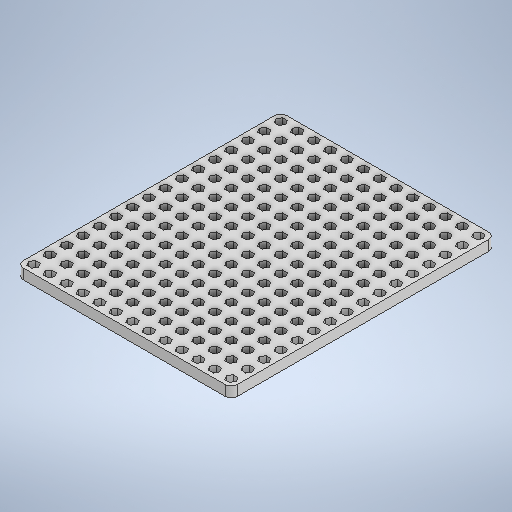
# Autodesk Inventor part: bottom
Saved by Autodesk Inventor 2025.1 (Build 291241000, 241)
## iProperties
Created: 2024-10-26
Part Number: bottom
Material: 일반
Document SubType Name: Sheet Metal
Designer: goode
Density: 1 g/cm^3
Sheet Metal Rule: 기본값_mm
Appearance: 기본값
Author: goode
Autodesk Inventor part; units mm, degrees
(part 1 of 2)
ref_plane "YZ Plane" through (0, 0, 0) normal (1, 0, 0) x (0, 1, 0)
ref_plane "XZ Plane" through (0, 0, 0) normal (0, 1, 0) x (-1, 0, 0)
ref_plane "XY Plane" through (0, 0, 0) normal (0, 0, 1) x (1, 0, 0)
sketch "스케치1" plane through (0, 0, 0) normal (0, 1, 0) x (-1, 0, 0)
  circle A0 centre (0, 0) radius 2.05
  line L0 (-1.1836, 2.05) -> (1.1836, 2.05)
  line L1 (1.1836, 2.05) -> (2.3671, 0)
  line L2 (2.3671, 0) -> (1.1836, -2.05)
  line L3 (1.1836, -2.05) -> (-1.1836, -2.05)
  line L4 (-1.1836, -2.05) -> (-2.3671, 0)
  line L5 (-2.3671, 0) -> (-1.1836, 2.05)
  circle A1 centre (0, 0) radius 1.1
  line L6 (-3, 0) -> (-3, 3)
  line L7 (-3, 3) -> (0, 3)
  circle A2 centre (0, -8) radius 2.05
  line L8 (-1.1836, -5.95) -> (1.1836, -5.95)
  line L9 (1.1836, -5.95) -> (2.3671, -8)
  line L10 (2.3671, -8) -> (1.1836, -10.05)
  line L11 (1.1836, -10.05) -> (-1.1836, -10.05)
  line L12 (-1.1836, -10.05) -> (-2.3671, -8)
  line L13 (-2.3671, -8) -> (-1.1836, -5.95)
  circle A3 centre (0, -8) radius 1.1
  circle A4 centre (0, -16) radius 2.05
  line L14 (-1.1836, -13.95) -> (1.1836, -13.95)
  line L15 (1.1836, -13.95) -> (2.3671, -16)
  line L16 (2.3671, -16) -> (1.1836, -18.05)
  line L17 (1.1836, -18.05) -> (-1.1836, -18.05)
  line L18 (-1.1836, -18.05) -> (-2.3671, -16)
  line L19 (-2.3671, -16) -> (-1.1836, -13.95)
  circle A5 centre (0, -16) radius 1.1
  circle A6 centre (0, -24) radius 2.05
  line L20 (-1.1836, -21.95) -> (1.1836, -21.95)
  line L21 (1.1836, -21.95) -> (2.3671, -24)
  line L22 (2.3671, -24) -> (1.1836, -26.05)
  line L23 (1.1836, -26.05) -> (-1.1836, -26.05)
  line L24 (-1.1836, -26.05) -> (-2.3671, -24)
  line L25 (-2.3671, -24) -> (-1.1836, -21.95)
  circle A7 centre (0, -24) radius 1.1
  circle A8 centre (0, -32) radius 2.05
  line L26 (-1.1836, -29.95) -> (1.1836, -29.95)
  line L27 (1.1836, -29.95) -> (2.3671, -32)
  line L28 (2.3671, -32) -> (1.1836, -34.05)
  line L29 (1.1836, -34.05) -> (-1.1836, -34.05)
  line L30 (-1.1836, -34.05) -> (-2.3671, -32)
  line L31 (-2.3671, -32) -> (-1.1836, -29.95)
  circle A9 centre (0, -32) radius 1.1
  circle A10 centre (0, -40) radius 2.05
  line L32 (-1.1836, -37.95) -> (1.1836, -37.95)
  line L33 (1.1836, -37.95) -> (2.3671, -40)
  line L34 (2.3671, -40) -> (1.1836, -42.05)
  line L35 (1.1836, -42.05) -> (-1.1836, -42.05)
  line L36 (-1.1836, -42.05) -> (-2.3671, -40)
  line L37 (-2.3671, -40) -> (-1.1836, -37.95)
  circle A11 centre (0, -40) radius 1.1
  circle A12 centre (0, -48) radius 2.05
  line L38 (-1.1836, -45.95) -> (1.1836, -45.95)
  line L39 (1.1836, -45.95) -> (2.3671, -48)
  line L40 (2.3671, -48) -> (1.1836, -50.05)
  line L41 (1.1836, -50.05) -> (-1.1836, -50.05)
  line L42 (-1.1836, -50.05) -> (-2.3671, -48)
  line L43 (-2.3671, -48) -> (-1.1836, -45.95)
  circle A13 centre (0, -48) radius 1.1
  circle A14 centre (0, -56) radius 2.05
  line L44 (-1.1836, -53.95) -> (1.1836, -53.95)
  line L45 (1.1836, -53.95) -> (2.3671, -56)
  line L46 (2.3671, -56) -> (1.1836, -58.05)
  line L47 (1.1836, -58.05) -> (-1.1836, -58.05)
  line L48 (-1.1836, -58.05) -> (-2.3671, -56)
  line L49 (-2.3671, -56) -> (-1.1836, -53.95)
  circle A15 centre (0, -56) radius 1.1
  circle A16 centre (0, -64) radius 2.05
  line L50 (-1.1836, -61.95) -> (1.1836, -61.95)
  line L51 (1.1836, -61.95) -> (2.3671, -64)
  line L52 (2.3671, -64) -> (1.1836, -66.05)
  line L53 (1.1836, -66.05) -> (-1.1836, -66.05)
  line L54 (-1.1836, -66.05) -> (-2.3671, -64)
  line L55 (-2.3671, -64) -> (-1.1836, -61.95)
  circle A17 centre (0, -64) radius 1.1
  circle A18 centre (0, -72) radius 2.05
  line L56 (-1.1836, -69.95) -> (1.1836, -69.95)
  line L57 (1.1836, -69.95) -> (2.3671, -72)
  line L58 (2.3671, -72) -> (1.1836, -74.05)
  line L59 (1.1836, -74.05) -> (-1.1836, -74.05)
  line L60 (-1.1836, -74.05) -> (-2.3671, -72)
  line L61 (-2.3671, -72) -> (-1.1836, -69.95)
  circle A19 centre (0, -72) radius 1.1
  circle A20 centre (0, -80) radius 2.05
  line L62 (-1.1836, -77.95) -> (1.1836, -77.95)
  line L63 (1.1836, -77.95) -> (2.3671, -80)
  line L64 (2.3671, -80) -> (1.1836, -82.05)
  line L65 (1.1836, -82.05) -> (-1.1836, -82.05)
  line L66 (-1.1836, -82.05) -> (-2.3671, -80)
  line L67 (-2.3671, -80) -> (-1.1836, -77.95)
  circle A21 centre (0, -80) radius 1.1
  circle A22 centre (0, -88) radius 2.05
  line L68 (-1.1836, -85.95) -> (1.1836, -85.95)
  line L69 (1.1836, -85.95) -> (2.3671, -88)
  line L70 (2.3671, -88) -> (1.1836, -90.05)
  line L71 (1.1836, -90.05) -> (-1.1836, -90.05)
  line L72 (-1.1836, -90.05) -> (-2.3671, -88)
  line L73 (-2.3671, -88) -> (-1.1836, -85.95)
  circle A23 centre (0, -88) radius 1.1
  circle A24 centre (0, -96) radius 2.05
  line L74 (-1.1836, -93.95) -> (1.1836, -93.95)
  line L75 (1.1836, -93.95) -> (2.3671, -96)
  line L76 (2.3671, -96) -> (1.1836, -98.05)
  line L77 (1.1836, -98.05) -> (-1.1836, -98.05)
  line L78 (-1.1836, -98.05) -> (-2.3671, -96)
  line L79 (-2.3671, -96) -> (-1.1836, -93.95)
  circle A25 centre (0, -96) radius 1.1
  circle A26 centre (0, -104) radius 2.05
  line L80 (-1.1836, -101.95) -> (1.1836, -101.95)
  line L81 (1.1836, -101.95) -> (2.3671, -104)
  line L82 (2.3671, -104) -> (1.1836, -106.05)
  line L83 (1.1836, -106.05) -> (-1.1836, -106.05)
  line L84 (-1.1836, -106.05) -> (-2.3671, -104)
  line L85 (-2.3671, -104) -> (-1.1836, -101.95)
  circle A27 centre (0, -104) radius 1.1
  circle A28 centre (0, -112) radius 2.05
  line L86 (-1.1836, -109.95) -> (1.1836, -109.95)
  line L87 (1.1836, -109.95) -> (2.3671, -112)
  line L88 (2.3671, -112) -> (1.1836, -114.05)
  line L89 (1.1836, -114.05) -> (-1.1836, -114.05)
  line L90 (-1.1836, -114.05) -> (-2.3671, -112)
  line L91 (-2.3671, -112) -> (-1.1836, -109.95)
  circle A29 centre (0, -112) radius 1.1
  circle A30 centre (0, -120) radius 2.05
  line L92 (-1.1836, -117.95) -> (1.1836, -117.95)
  line L93 (1.1836, -117.95) -> (2.3671, -120)
  line L94 (2.3671, -120) -> (1.1836, -122.05)
  line L95 (1.1836, -122.05) -> (-1.1836, -122.05)
  line L96 (-1.1836, -122.05) -> (-2.3671, -120)
  line L97 (-2.3671, -120) -> (-1.1836, -117.95)
  circle A31 centre (0, -120) radius 1.1
  circle A32 centre (8, 0) radius 2.05
  line L98 (6.8164, 2.05) -> (9.1836, 2.05)
  line L99 (9.1836, 2.05) -> (10.3671, 0)
  line L100 (10.3671, 0) -> (9.1836, -2.05)
  line L101 (9.1836, -2.05) -> (6.8164, -2.05)
  line L102 (6.8164, -2.05) -> (5.6329, 0)
  line L103 (5.6329, 0) -> (6.8164, 2.05)
  circle A33 centre (8, 0) radius 1.1
  circle A34 centre (8, -8) radius 2.05
  line L104 (6.8164, -5.95) -> (9.1836, -5.95)
  line L105 (9.1836, -5.95) -> (10.3671, -8)
  line L106 (10.3671, -8) -> (9.1836, -10.05)
  line L107 (9.1836, -10.05) -> (6.8164, -10.05)
  line L108 (6.8164, -10.05) -> (5.6329, -8)
  line L109 (5.6329, -8) -> (6.8164, -5.95)
  circle A35 centre (8, -8) radius 1.1
  circle A36 centre (8, -16) radius 2.05
  line L110 (6.8164, -13.95) -> (9.1836, -13.95)
  line L111 (9.1836, -13.95) -> (10.3671, -16)
  line L112 (10.3671, -16) -> (9.1836, -18.05)
  line L113 (9.1836, -18.05) -> (6.8164, -18.05)
  line L114 (6.8164, -18.05) -> (5.6329, -16)
  line L115 (5.6329, -16) -> (6.8164, -13.95)
  circle A37 centre (8, -16) radius 1.1
  circle A38 centre (8, -24) radius 2.05
  line L116 (6.8164, -21.95) -> (9.1836, -21.95)
  line L117 (9.1836, -21.95) -> (10.3671, -24)
  line L118 (10.3671, -24) -> (9.1836, -26.05)
  line L119 (9.1836, -26.05) -> (6.8164, -26.05)
  line L120 (6.8164, -26.05) -> (5.6329, -24)
  line L121 (5.6329, -24) -> (6.8164, -21.95)
  circle A39 centre (8, -24) radius 1.1
  circle A40 centre (8, -32) radius 2.05
  line L122 (6.8164, -29.95) -> (9.1836, -29.95)
  line L123 (9.1836, -29.95) -> (10.3671, -32)
  line L124 (10.3671, -32) -> (9.1836, -34.05)
  line L125 (9.1836, -34.05) -> (6.8164, -34.05)
  line L126 (6.8164, -34.05) -> (5.6329, -32)
  line L127 (5.6329, -32) -> (6.8164, -29.95)
  circle A41 centre (8, -32) radius 1.1
  circle A42 centre (8, -40) radius 2.05
  line L128 (6.8164, -37.95) -> (9.1836, -37.95)
  line L129 (9.1836, -37.95) -> (10.3671, -40)
  line L130 (10.3671, -40) -> (9.1836, -42.05)
  line L131 (9.1836, -42.05) -> (6.8164, -42.05)
  line L132 (6.8164, -42.05) -> (5.6329, -40)
  line L133 (5.6329, -40) -> (6.8164, -37.95)
  circle A43 centre (8, -40) radius 1.1
  circle A44 centre (8, -48) radius 2.05
  line L134 (6.8164, -45.95) -> (9.1836, -45.95)
  line L135 (9.1836, -45.95) -> (10.3671, -48)
  line L136 (10.3671, -48) -> (9.1836, -50.05)
  line L137 (9.1836, -50.05) -> (6.8164, -50.05)
  line L138 (6.8164, -50.05) -> (5.6329, -48)
  line L139 (5.6329, -48) -> (6.8164, -45.95)
  circle A45 centre (8, -48) radius 1.1
  circle A46 centre (8, -56) radius 2.05
  line L140 (6.8164, -53.95) -> (9.1836, -53.95)
  line L141 (9.1836, -53.95) -> (10.3671, -56)
  line L142 (10.3671, -56) -> (9.1836, -58.05)
  line L143 (9.1836, -58.05) -> (6.8164, -58.05)
  line L144 (6.8164, -58.05) -> (5.6329, -56)
  line L145 (5.6329, -56) -> (6.8164, -53.95)
  circle A47 centre (8, -56) radius 1.1
  circle A48 centre (8, -64) radius 2.05
  line L146 (6.8164, -61.95) -> (9.1836, -61.95)
  line L147 (9.1836, -61.95) -> (10.3671, -64)
  line L148 (10.3671, -64) -> (9.1836, -66.05)
  line L149 (9.1836, -66.05) -> (6.8164, -66.05)
  line L150 (6.8164, -66.05) -> (5.6329, -64)
  line L151 (5.6329, -64) -> (6.8164, -61.95)
  circle A49 centre (8, -64) radius 1.1
  circle A50 centre (8, -72) radius 2.05
  line L152 (6.8164, -69.95) -> (9.1836, -69.95)
  line L153 (9.1836, -69.95) -> (10.3671, -72)
  line L154 (10.3671, -72) -> (9.1836, -74.05)
  line L155 (9.1836, -74.05) -> (6.8164, -74.05)
  line L156 (6.8164, -74.05) -> (5.6329, -72)
  line L157 (5.6329, -72) -> (6.8164, -69.95)
  circle A51 centre (8, -72) radius 1.1
  circle A52 centre (8, -80) radius 2.05
  line L158 (6.8164, -77.95) -> (9.1836, -77.95)
  line L159 (9.1836, -77.95) -> (10.3671, -80)
  line L160 (10.3671, -80) -> (9.1836, -82.05)
  line L161 (9.1836, -82.05) -> (6.8164, -82.05)
  line L162 (6.8164, -82.05) -> (5.6329, -80)
  line L163 (5.6329, -80) -> (6.8164, -77.95)
  circle A53 centre (8, -80) radius 1.1
  circle A54 centre (8, -88) radius 2.05
  line L164 (6.8164, -85.95) -> (9.1836, -85.95)
  line L165 (9.1836, -85.95) -> (10.3671, -88)
  line L166 (10.3671, -88) -> (9.1836, -90.05)
  line L167 (9.1836, -90.05) -> (6.8164, -90.05)
  line L168 (6.8164, -90.05) -> (5.6329, -88)
  line L169 (5.6329, -88) -> (6.8164, -85.95)
  circle A55 centre (8, -88) radius 1.1
  circle A56 centre (8, -96) radius 2.05
  line L170 (6.8164, -93.95) -> (9.1836, -93.95)
  line L171 (9.1836, -93.95) -> (10.3671, -96)
  line L172 (10.3671, -96) -> (9.1836, -98.05)
  line L173 (9.1836, -98.05) -> (6.8164, -98.05)
  line L174 (6.8164, -98.05) -> (5.6329, -96)
  line L175 (5.6329, -96) -> (6.8164, -93.95)
  circle A57 centre (8, -96) radius 1.1
  circle A58 centre (8, -104) radius 2.05
  line L176 (6.8164, -101.95) -> (9.1836, -101.95)
  line L177 (9.1836, -101.95) -> (10.3671, -104)
  line L178 (10.3671, -104) -> (9.1836, -106.05)
  line L179 (9.1836, -106.05) -> (6.8164, -106.05)
  line L180 (6.8164, -106.05) -> (5.6329, -104)
  line L181 (5.6329, -104) -> (6.8164, -101.95)
  circle A59 centre (8, -104) radius 1.1
  circle A60 centre (8, -112) radius 2.05
  line L182 (6.8164, -109.95) -> (9.1836, -109.95)
  line L183 (9.1836, -109.95) -> (10.3671, -112)
  line L184 (10.3671, -112) -> (9.1836, -114.05)
  line L185 (9.1836, -114.05) -> (6.8164, -114.05)
  line L186 (6.8164, -114.05) -> (5.6329, -112)
  line L187 (5.6329, -112) -> (6.8164, -109.95)
  circle A61 centre (8, -112) radius 1.1
  circle A62 centre (8, -120) radius 2.05
  line L188 (6.8164, -117.95) -> (9.1836, -117.95)
  line L189 (9.1836, -117.95) -> (10.3671, -120)
  line L190 (10.3671, -120) -> (9.1836, -122.05)
  line L191 (9.1836, -122.05) -> (6.8164, -122.05)
  line L192 (6.8164, -122.05) -> (5.6329, -120)
  line L193 (5.6329, -120) -> (6.8164, -117.95)
  circle A63 centre (8, -120) radius 1.1
  circle A64 centre (16, 0) radius 2.05
  line L194 (14.8164, 2.05) -> (17.1836, 2.05)
  line L195 (17.1836, 2.05) -> (18.3671, 0)
  line L196 (18.3671, 0) -> (17.1836, -2.05)
  line L197 (17.1836, -2.05) -> (14.8164, -2.05)
  line L198 (14.8164, -2.05) -> (13.6329, 0)
  line L199 (13.6329, 0) -> (14.8164, 2.05)
  circle A65 centre (16, 0) radius 1.1
  circle A66 centre (16, -8) radius 2.05
  line L200 (14.8164, -5.95) -> (17.1836, -5.95)
  line L201 (17.1836, -5.95) -> (18.3671, -8)
  line L202 (18.3671, -8) -> (17.1836, -10.05)
  line L203 (17.1836, -10.05) -> (14.8164, -10.05)
  line L204 (14.8164, -10.05) -> (13.6329, -8)
  line L205 (13.6329, -8) -> (14.8164, -5.95)
  circle A67 centre (16, -8) radius 1.1
  circle A68 centre (16, -16) radius 2.05
  line L206 (14.8164, -13.95) -> (17.1836, -13.95)
  line L207 (17.1836, -13.95) -> (18.3671, -16)
  line L208 (18.3671, -16) -> (17.1836, -18.05)
  line L209 (17.1836, -18.05) -> (14.8164, -18.05)
  line L210 (14.8164, -18.05) -> (13.6329, -16)
  line L211 (13.6329, -16) -> (14.8164, -13.95)
  circle A69 centre (16, -16) radius 1.1
  circle A70 centre (16, -24) radius 2.05
  line L212 (14.8164, -21.95) -> (17.1836, -21.95)
  line L213 (17.1836, -21.95) -> (18.3671, -24)
  line L214 (18.3671, -24) -> (17.1836, -26.05)
  line L215 (17.1836, -26.05) -> (14.8164, -26.05)
  line L216 (14.8164, -26.05) -> (13.6329, -24)
  line L217 (13.6329, -24) -> (14.8164, -21.95)
  circle A71 centre (16, -24) radius 1.1
  circle A72 centre (16, -32) radius 2.05
  line L218 (14.8164, -29.95) -> (17.1836, -29.95)
  line L219 (17.1836, -29.95) -> (18.3671, -32)
  line L220 (18.3671, -32) -> (17.1836, -34.05)
  line L221 (17.1836, -34.05) -> (14.8164, -34.05)
  line L222 (14.8164, -34.05) -> (13.6329, -32)
  line L223 (13.6329, -32) -> (14.8164, -29.95)
  circle A73 centre (16, -32) radius 1.1
  circle A74 centre (16, -40) radius 2.05
  line L224 (14.8164, -37.95) -> (17.1836, -37.95)
  line L225 (17.1836, -37.95) -> (18.3671, -40)
  line L226 (18.3671, -40) -> (17.1836, -42.05)
  line L227 (17.1836, -42.05) -> (14.8164, -42.05)
  line L228 (14.8164, -42.05) -> (13.6329, -40)
  line L229 (13.6329, -40) -> (14.8164, -37.95)
  circle A75 centre (16, -40) radius 1.1
  circle A76 centre (16, -48) radius 2.05
  line L230 (14.8164, -45.95) -> (17.1836, -45.95)
  line L231 (17.1836, -45.95) -> (18.3671, -48)
  line L232 (18.3671, -48) -> (17.1836, -50.05)
  line L233 (17.1836, -50.05) -> (14.8164, -50.05)
  line L234 (14.8164, -50.05) -> (13.6329, -48)
  line L235 (13.6329, -48) -> (14.8164, -45.95)
  circle A77 centre (16, -48) radius 1.1
  circle A78 centre (16, -56) radius 2.05
  line L236 (14.8164, -53.95) -> (17.1836, -53.95)
  line L237 (17.1836, -53.95) -> (18.3671, -56)
  line L238 (18.3671, -56) -> (17.1836, -58.05)
  line L239 (17.1836, -58.05) -> (14.8164, -58.05)
  line L240 (14.8164, -58.05) -> (13.6329, -56)
  line L241 (13.6329, -56) -> (14.8164, -53.95)
  circle A79 centre (16, -56) radius 1.1
  circle A80 centre (16, -64) radius 2.05
  line L242 (14.8164, -61.95) -> (17.1836, -61.95)
  line L243 (17.1836, -61.95) -> (18.3671, -64)
  line L244 (18.3671, -64) -> (17.1836, -66.05)
  line L245 (17.1836, -66.05) -> (14.8164, -66.05)
  line L246 (14.8164, -66.05) -> (13.6329, -64)
  line L247 (13.6329, -64) -> (14.8164, -61.95)
  circle A81 centre (16, -64) radius 1.1
  circle A82 centre (16, -72) radius 2.05
  line L248 (14.8164, -69.95) -> (17.1836, -69.95)
  line L249 (17.1836, -69.95) -> (18.3671, -72)
  line L250 (18.3671, -72) -> (17.1836, -74.05)
  line L251 (17.1836, -74.05) -> (14.8164, -74.05)
  line L252 (14.8164, -74.05) -> (13.6329, -72)
  line L253 (13.6329, -72) -> (14.8164, -69.95)
  circle A83 centre (16, -72) radius 1.1
  circle A84 centre (16, -80) radius 2.05
  line L254 (14.8164, -77.95) -> (17.1836, -77.95)
  line L255 (17.1836, -77.95) -> (18.3671, -80)
  line L256 (18.3671, -80) -> (17.1836, -82.05)
  line L257 (17.1836, -82.05) -> (14.8164, -82.05)
  line L258 (14.8164, -82.05) -> (13.6329, -80)
  line L259 (13.6329, -80) -> (14.8164, -77.95)
  circle A85 centre (16, -80) radius 1.1
  circle A86 centre (16, -88) radius 2.05
  line L260 (14.8164, -85.95) -> (17.1836, -85.95)
  line L261 (17.1836, -85.95) -> (18.3671, -88)
  line L262 (18.3671, -88) -> (17.1836, -90.05)
  line L263 (17.1836, -90.05) -> (14.8164, -90.05)
  line L264 (14.8164, -90.05) -> (13.6329, -88)
  line L265 (13.6329, -88) -> (14.8164, -85.95)
  circle A87 centre (16, -88) radius 1.1
  circle A88 centre (16, -96) radius 2.05
  line L266 (14.8164, -93.95) -> (17.1836, -93.95)
  line L267 (17.1836, -93.95) -> (18.3671, -96)
  line L268 (18.3671, -96) -> (17.1836, -98.05)
  line L269 (17.1836, -98.05) -> (14.8164, -98.05)
  line L270 (14.8164, -98.05) -> (13.6329, -96)
  line L271 (13.6329, -96) -> (14.8164, -93.95)
  circle A89 centre (16, -96) radius 1.1
  circle A90 centre (16, -104) radius 2.05
  line L272 (14.8164, -101.95) -> (17.1836, -101.95)
  line L273 (17.1836, -101.95) -> (18.3671, -104)
  line L274 (18.3671, -104) -> (17.1836, -106.05)
  line L275 (17.1836, -106.05) -> (14.8164, -106.05)
  line L276 (14.8164, -106.05) -> (13.6329, -104)
  line L277 (13.6329, -104) -> (14.8164, -101.95)
  circle A91 centre (16, -104) radius 1.1
  circle A92 centre (16, -112) radius 2.05
  line L278 (14.8164, -109.95) -> (17.1836, -109.95)
  line L279 (17.1836, -109.95) -> (18.3671, -112)
  line L280 (18.3671, -112) -> (17.1836, -114.05)
  line L281 (17.1836, -114.05) -> (14.8164, -114.05)
  line L282 (14.8164, -114.05) -> (13.6329, -112)
  line L283 (13.6329, -112) -> (14.8164, -109.95)
  circle A93 centre (16, -112) radius 1.1
  circle A94 centre (16, -120) radius 2.05
  line L284 (14.8164, -117.95) -> (17.1836, -117.95)
  line L285 (17.1836, -117.95) -> (18.3671, -120)
  line L286 (18.3671, -120) -> (17.1836, -122.05)
  line L287 (17.1836, -122.05) -> (14.8164, -122.05)
  line L288 (14.8164, -122.05) -> (13.6329, -120)
  line L289 (13.6329, -120) -> (14.8164, -117.95)
  circle A95 centre (16, -120) radius 1.1
  circle A96 centre (24, 0) radius 2.05
  line L290 (22.8164, 2.05) -> (25.1836, 2.05)
  line L291 (25.1836, 2.05) -> (26.3671, 0)
  line L292 (26.3671, 0) -> (25.1836, -2.05)
  line L293 (25.1836, -2.05) -> (22.8164, -2.05)
  line L294 (22.8164, -2.05) -> (21.6329, 0)
  line L295 (21.6329, 0) -> (22.8164, 2.05)
  circle A97 centre (24, 0) radius 1.1
  circle A98 centre (24, -8) radius 2.05
  line L296 (22.8164, -5.95) -> (25.1836, -5.95)
  line L297 (25.1836, -5.95) -> (26.3671, -8)
  line L298 (26.3671, -8) -> (25.1836, -10.05)
  line L299 (25.1836, -10.05) -> (22.8164, -10.05)
  line L300 (22.8164, -10.05) -> (21.6329, -8)
  line L301 (21.6329, -8) -> (22.8164, -5.95)
  circle A99 centre (24, -8) radius 1.1
  circle A100 centre (24, -16) radius 2.05
  line L302 (22.8164, -13.95) -> (25.1836, -13.95)
  line L303 (25.1836, -13.95) -> (26.3671, -16)
  line L304 (26.3671, -16) -> (25.1836, -18.05)
  line L305 (25.1836, -18.05) -> (22.8164, -18.05)
  line L306 (22.8164, -18.05) -> (21.6329, -16)
  line L307 (21.6329, -16) -> (22.8164, -13.95)
  circle A101 centre (24, -16) radius 1.1
  circle A102 centre (24, -24) radius 2.05
  line L308 (22.8164, -21.95) -> (25.1836, -21.95)
  line L309 (25.1836, -21.95) -> (26.3671, -24)
  line L310 (26.3671, -24) -> (25.1836, -26.05)
  line L311 (25.1836, -26.05) -> (22.8164, -26.05)
  line L312 (22.8164, -26.05) -> (21.6329, -24)
  line L313 (21.6329, -24) -> (22.8164, -21.95)
  circle A103 centre (24, -24) radius 1.1
  circle A104 centre (24, -32) radius 2.05
  line L314 (22.8164, -29.95) -> (25.1836, -29.95)
  line L315 (25.1836, -29.95) -> (26.3671, -32)
  line L316 (26.3671, -32) -> (25.1836, -34.05)
  line L317 (25.1836, -34.05) -> (22.8164, -34.05)
  line L318 (22.8164, -34.05) -> (21.6329, -32)
  line L319 (21.6329, -32) -> (22.8164, -29.95)
  circle A105 centre (24, -32) radius 1.1
  circle A106 centre (24, -40) radius 2.05
  line L320 (22.8164, -37.95) -> (25.1836, -37.95)
  line L321 (25.1836, -37.95) -> (26.3671, -40)
  line L322 (26.3671, -40) -> (25.1836, -42.05)
  line L323 (25.1836, -42.05) -> (22.8164, -42.05)
  line L324 (22.8164, -42.05) -> (21.6329, -40)
  line L325 (21.6329, -40) -> (22.8164, -37.95)
  circle A107 centre (24, -40) radius 1.1
  circle A108 centre (24, -48) radius 2.05
  line L326 (22.8164, -45.95) -> (25.1836, -45.95)
  line L327 (25.1836, -45.95) -> (26.3671, -48)
  line L328 (26.3671, -48) -> (25.1836, -50.05)
  line L329 (25.1836, -50.05) -> (22.8164, -50.05)
  line L330 (22.8164, -50.05) -> (21.6329, -48)
  line L331 (21.6329, -48) -> (22.8164, -45.95)
  circle A109 centre (24, -48) radius 1.1
  circle A110 centre (24, -56) radius 2.05
  line L332 (22.8164, -53.95) -> (25.1836, -53.95)
  line L333 (25.1836, -53.95) -> (26.3671, -56)
  line L334 (26.3671, -56) -> (25.1836, -58.05)
  line L335 (25.1836, -58.05) -> (22.8164, -58.05)
  line L336 (22.8164, -58.05) -> (21.6329, -56)
  line L337 (21.6329, -56) -> (22.8164, -53.95)
  circle A111 centre (24, -56) radius 1.1
  circle A112 centre (24, -64) radius 2.05
  line L338 (22.8164, -61.95) -> (25.1836, -61.95)
  line L339 (25.1836, -61.95) -> (26.3671, -64)
  line L340 (26.3671, -64) -> (25.1836, -66.05)
  line L341 (25.1836, -66.05) -> (22.8164, -66.05)
  line L342 (22.8164, -66.05) -> (21.6329, -64)
  line L343 (21.6329, -64) -> (22.8164, -61.95)
  circle A113 centre (24, -64) radius 1.1
  circle A114 centre (24, -72) radius 2.05
  line L344 (22.8164, -69.95) -> (25.1836, -69.95)
  line L345 (25.1836, -69.95) -> (26.3671, -72)
  line L346 (26.3671, -72) -> (25.1836, -74.05)
  line L347 (25.1836, -74.05) -> (22.8164, -74.05)
  line L348 (22.8164, -74.05) -> (21.6329, -72)
  line L349 (21.6329, -72) -> (22.8164, -69.95)
  circle A115 centre (24, -72) radius 1.1
  circle A116 centre (24, -80) radius 2.05
  line L350 (22.8164, -77.95) -> (25.1836, -77.95)
  line L351 (25.1836, -77.95) -> (26.3671, -80)
  line L352 (26.3671, -80) -> (25.1836, -82.05)
  line L353 (25.1836, -82.05) -> (22.8164, -82.05)
  line L354 (22.8164, -82.05) -> (21.6329, -80)
  line L355 (21.6329, -80) -> (22.8164, -77.95)
  circle A117 centre (24, -80) radius 1.1
  circle A118 centre (24, -88) radius 2.05
  line L356 (22.8164, -85.95) -> (25.1836, -85.95)
  line L357 (25.1836, -85.95) -> (26.3671, -88)
  line L358 (26.3671, -88) -> (25.1836, -90.05)
  line L359 (25.1836, -90.05) -> (22.8164, -90.05)
  line L360 (22.8164, -90.05) -> (21.6329, -88)
  line L361 (21.6329, -88) -> (22.8164, -85.95)
  circle A119 centre (24, -88) radius 1.1
  circle A120 centre (24, -96) radius 2.05
  line L362 (22.8164, -93.95) -> (25.1836, -93.95)
  line L363 (25.1836, -93.95) -> (26.3671, -96)
  line L364 (26.3671, -96) -> (25.1836, -98.05)
  line L365 (25.1836, -98.05) -> (22.8164, -98.05)
  line L366 (22.8164, -98.05) -> (21.6329, -96)
  line L367 (21.6329, -96) -> (22.8164, -93.95)
  circle A121 centre (24, -96) radius 1.1
  circle A122 centre (24, -104) radius 2.05
  line L368 (22.8164, -101.95) -> (25.1836, -101.95)
  line L369 (25.1836, -101.95) -> (26.3671, -104)
  line L370 (26.3671, -104) -> (25.1836, -106.05)
  line L371 (25.1836, -106.05) -> (22.8164, -106.05)
  line L372 (22.8164, -106.05) -> (21.6329, -104)
  line L373 (21.6329, -104) -> (22.8164, -101.95)
  circle A123 centre (24, -104) radius 1.1
  circle A124 centre (24, -112) radius 2.05
  line L374 (22.8164, -109.95) -> (25.1836, -109.95)
  line L375 (25.1836, -109.95) -> (26.3671, -112)
  line L376 (26.3671, -112) -> (25.1836, -114.05)
  line L377 (25.1836, -114.05) -> (22.8164, -114.05)
  line L378 (22.8164, -114.05) -> (21.6329, -112)
  line L379 (21.6329, -112) -> (22.8164, -109.95)
  circle A125 centre (24, -112) radius 1.1
  circle A126 centre (24, -120) radius 2.05
  line L380 (22.8164, -117.95) -> (25.1836, -117.95)
  line L381 (25.1836, -117.95) -> (26.3671, -120)
  line L382 (26.3671, -120) -> (25.1836, -122.05)
  line L383 (25.1836, -122.05) -> (22.8164, -122.05)
  line L384 (22.8164, -122.05) -> (21.6329, -120)
  line L385 (21.6329, -120) -> (22.8164, -117.95)
  circle A127 centre (24, -120) radius 1.1
  circle A128 centre (32, 0) radius 2.05
  line L386 (30.8164, 2.05) -> (33.1836, 2.05)
  line L387 (33.1836, 2.05) -> (34.3671, 0)
  line L388 (34.3671, 0) -> (33.1836, -2.05)
  line L389 (33.1836, -2.05) -> (30.8164, -2.05)
  line L390 (30.8164, -2.05) -> (29.6329, 0)
  line L391 (29.6329, 0) -> (30.8164, 2.05)
  circle A129 centre (32, 0) radius 1.1
  circle A130 centre (32, -8) radius 2.05
  line L392 (30.8164, -5.95) -> (33.1836, -5.95)
  line L393 (33.1836, -5.95) -> (34.3671, -8)
  line L394 (34.3671, -8) -> (33.1836, -10.05)
  line L395 (33.1836, -10.05) -> (30.8164, -10.05)
  line L396 (30.8164, -10.05) -> (29.6329, -8)
  line L397 (29.6329, -8) -> (30.8164, -5.95)
  circle A131 centre (32, -8) radius 1.1
  circle A132 centre (32, -16) radius 2.05
  line L398 (30.8164, -13.95) -> (33.1836, -13.95)
  line L399 (33.1836, -13.95) -> (34.3671, -16)
  line L400 (34.3671, -16) -> (33.1836, -18.05)
  line L401 (33.1836, -18.05) -> (30.8164, -18.05)
  line L402 (30.8164, -18.05) -> (29.6329, -16)
  line L403 (29.6329, -16) -> (30.8164, -13.95)
  circle A133 centre (32, -16) radius 1.1
  circle A134 centre (32, -24) radius 2.05
  line L404 (30.8164, -21.95) -> (33.1836, -21.95)
  line L405 (33.1836, -21.95) -> (34.3671, -24)
  line L406 (34.3671, -24) -> (33.1836, -26.05)
  line L407 (33.1836, -26.05) -> (30.8164, -26.05)
  line L408 (30.8164, -26.05) -> (29.6329, -24)
  line L409 (29.6329, -24) -> (30.8164, -21.95)
  circle A135 centre (32, -24) radius 1.1
  circle A136 centre (32, -32) radius 2.05
  line L410 (30.8164, -29.95) -> (33.1836, -29.95)
  line L411 (33.1836, -29.95) -> (34.3671, -32)
  line L412 (34.3671, -32) -> (33.1836, -34.05)
  line L413 (33.1836, -34.05) -> (30.8164, -34.05)
  line L414 (30.8164, -34.05) -> (29.6329, -32)
  line L415 (29.6329, -32) -> (30.8164, -29.95)
  circle A137 centre (32, -32) radius 1.1
  circle A138 centre (32, -40) radius 2.05
  line L416 (30.8164, -37.95) -> (33.1836, -37.95)
  line L417 (33.1836, -37.95) -> (34.3671, -40)
  line L418 (34.3671, -40) -> (33.1836, -42.05)
  line L419 (33.1836, -42.05) -> (30.8164, -42.05)
  line L420 (30.8164, -42.05) -> (29.6329, -40)
  line L421 (29.6329, -40) -> (30.8164, -37.95)
  circle A139 centre (32, -40) radius 1.1
  circle A140 centre (32, -48) radius 2.05
  line L422 (30.8164, -45.95) -> (33.1836, -45.95)
  line L423 (33.1836, -45.95) -> (34.3671, -48)
  line L424 (34.3671, -48) -> (33.1836, -50.05)
  line L425 (33.1836, -50.05) -> (30.8164, -50.05)
  line L426 (30.8164, -50.05) -> (29.6329, -48)
  line L427 (29.6329, -48) -> (30.8164, -45.95)
  circle A141 centre (32, -48) radius 1.1
  circle A142 centre (32, -56) radius 2.05
  line L428 (30.8164, -53.95) -> (33.1836, -53.95)
  line L429 (33.1836, -53.95) -> (34.3671, -56)
  line L430 (34.3671, -56) -> (33.1836, -58.05)
  line L431 (33.1836, -58.05) -> (30.8164, -58.05)
  line L432 (30.8164, -58.05) -> (29.6329, -56)
  line L433 (29.6329, -56) -> (30.8164, -53.95)
  circle A143 centre (32, -56) radius 1.1
  circle A144 centre (32, -64) radius 2.05
  line L434 (30.8164, -61.95) -> (33.1836, -61.95)
  line L435 (33.1836, -61.95) -> (34.3671, -64)
  line L436 (34.3671, -64) -> (33.1836, -66.05)
  line L437 (33.1836, -66.05) -> (30.8164, -66.05)
  line L438 (30.8164, -66.05) -> (29.6329, -64)
  line L439 (29.6329, -64) -> (30.8164, -61.95)
  circle A145 centre (32, -64) radius 1.1
  circle A146 centre (32, -72) radius 2.05
  line L440 (30.8164, -69.95) -> (33.1836, -69.95)
  line L441 (33.1836, -69.95) -> (34.3671, -72)
  line L442 (34.3671, -72) -> (33.1836, -74.05)
  line L443 (33.1836, -74.05) -> (30.8164, -74.05)
  line L444 (30.8164, -74.05) -> (29.6329, -72)
  line L445 (29.6329, -72) -> (30.8164, -69.95)
  circle A147 centre (32, -72) radius 1.1
  circle A148 centre (32, -80) radius 2.05
  line L446 (30.8164, -77.95) -> (33.1836, -77.95)
  line L447 (33.1836, -77.95) -> (34.3671, -80)
  line L448 (34.3671, -80) -> (33.1836, -82.05)
  line L449 (33.1836, -82.05) -> (30.8164, -82.05)
  line L450 (30.8164, -82.05) -> (29.6329, -80)
  line L451 (29.6329, -80) -> (30.8164, -77.95)
  circle A149 centre (32, -80) radius 1.1
  circle A150 centre (32, -88) radius 2.05
  line L452 (30.8164, -85.95) -> (33.1836, -85.95)
  line L453 (33.1836, -85.95) -> (34.3671, -88)
  line L454 (34.3671, -88) -> (33.1836, -90.05)
  line L455 (33.1836, -90.05) -> (30.8164, -90.05)
  line L456 (30.8164, -90.05) -> (29.6329, -88)
  line L457 (29.6329, -88) -> (30.8164, -85.95)
  circle A151 centre (32, -88) radius 1.1
  circle A152 centre (32, -96) radius 2.05
  line L458 (30.8164, -93.95) -> (33.1836, -93.95)
  line L459 (33.1836, -93.95) -> (34.3671, -96)
  line L460 (34.3671, -96) -> (33.1836, -98.05)
  line L461 (33.1836, -98.05) -> (30.8164, -98.05)
  line L462 (30.8164, -98.05) -> (29.6329, -96)
  line L463 (29.6329, -96) -> (30.8164, -93.95)
  circle A153 centre (32, -96) radius 1.1
  circle A154 centre (32, -104) radius 2.05
  line L464 (30.8164, -101.95) -> (33.1836, -101.95)
  line L465 (33.1836, -101.95) -> (34.3671, -104)
  line L466 (34.3671, -104) -> (33.1836, -106.05)
  line L467 (33.1836, -106.05) -> (30.8164, -106.05)
  line L468 (30.8164, -106.05) -> (29.6329, -104)
  line L469 (29.6329, -104) -> (30.8164, -101.95)
  circle A155 centre (32, -104) radius 1.1
  circle A156 centre (32, -112) radius 2.05
  line L470 (30.8164, -109.95) -> (33.1836, -109.95)
  line L471 (33.1836, -109.95) -> (34.3671, -112)
  line L472 (34.3671, -112) -> (33.1836, -114.05)
  line L473 (33.1836, -114.05) -> (30.8164, -114.05)
  line L474 (30.8164, -114.05) -> (29.6329, -112)
  line L475 (29.6329, -112) -> (30.8164, -109.95)
  circle A157 centre (32, -112) radius 1.1
  circle A158 centre (32, -120) radius 2.05
  line L476 (30.8164, -117.95) -> (33.1836, -117.95)
  line L477 (33.1836, -117.95) -> (34.3671, -120)
  line L478 (34.3671, -120) -> (33.1836, -122.05)
  line L479 (33.1836, -122.05) -> (30.8164, -122.05)
  line L480 (30.8164, -122.05) -> (29.6329, -120)
  line L481 (29.6329, -120) -> (30.8164, -117.95)
  circle A159 centre (32, -120) radius 1.1
  circle A160 centre (40, 0) radius 2.05
  line L482 (38.8164, 2.05) -> (41.1836, 2.05)
  line L483 (41.1836, 2.05) -> (42.3671, 0)
  line L484 (42.3671, 0) -> (41.1836, -2.05)
  line L485 (41.1836, -2.05) -> (38.8164, -2.05)
  line L486 (38.8164, -2.05) -> (37.6329, 0)
  line L487 (37.6329, 0) -> (38.8164, 2.05)
  circle A161 centre (40, 0) radius 1.1
  circle A162 centre (40, -8) radius 2.05
  line L488 (38.8164, -5.95) -> (41.1836, -5.95)
  line L489 (41.1836, -5.95) -> (42.3671, -8)
  line L490 (42.3671, -8) -> (41.1836, -10.05)
  line L491 (41.1836, -10.05) -> (38.8164, -10.05)
  line L492 (38.8164, -10.05) -> (37.6329, -8)
  line L493 (37.6329, -8) -> (38.8164, -5.95)
  circle A163 centre (40, -8) radius 1.1
  circle A164 centre (40, -16) radius 2.05
  line L494 (38.8164, -13.95) -> (41.1836, -13.95)
  line L495 (41.1836, -13.95) -> (42.3671, -16)
  line L496 (42.3671, -16) -> (41.1836, -18.05)
  line L497 (41.1836, -18.05) -> (38.8164, -18.05)
  line L498 (38.8164, -18.05) -> (37.6329, -16)
  line L499 (37.6329, -16) -> (38.8164, -13.95)
  circle A165 centre (40, -16) radius 1.1
  circle A166 centre (40, -24) radius 2.05
  line L500 (38.8164, -21.95) -> (41.1836, -21.95)
  line L501 (41.1836, -21.95) -> (42.3671, -24)
  line L502 (42.3671, -24) -> (41.1836, -26.05)
  line L503 (41.1836, -26.05) -> (38.8164, -26.05)
  line L504 (38.8164, -26.05) -> (37.6329, -24)
  line L505 (37.6329, -24) -> (38.8164, -21.95)
  circle A167 centre (40, -24) radius 1.1
  circle A168 centre (40, -32) radius 2.05
  line L506 (38.8164, -29.95) -> (41.1836, -29.95)
  line L507 (41.1836, -29.95) -> (42.3671, -32)
  line L508 (42.3671, -32) -> (41.1836, -34.05)
  line L509 (41.1836, -34.05) -> (38.8164, -34.05)
  line L510 (38.8164, -34.05) -> (37.6329, -32)
  line L511 (37.6329, -32) -> (38.8164, -29.95)
  circle A169 centre (40, -32) radius 1.1
  circle A170 centre (40, -40) radius 2.05
  line L512 (38.8164, -37.95) -> (41.1836, -37.95)
  line L513 (41.1836, -37.95) -> (42.3671, -40)
  line L514 (42.3671, -40) -> (41.1836, -42.05)
  line L515 (41.1836, -42.05) -> (38.8164, -42.05)
  line L516 (38.8164, -42.05) -> (37.6329, -40)
  line L517 (37.6329, -40) -> (38.8164, -37.95)
  circle A171 centre (40, -40) radius 1.1
  circle A172 centre (40, -48) radius 2.05
  line L518 (38.8164, -45.95) -> (41.1836, -45.95)
  line L519 (41.1836, -45.95) -> (42.3671, -48)
  line L520 (42.3671, -48) -> (41.1836, -50.05)
  line L521 (41.1836, -50.05) -> (38.8164, -50.05)
  line L522 (38.8164, -50.05) -> (37.6329, -48)
  line L523 (37.6329, -48) -> (38.8164, -45.95)
  circle A173 centre (40, -48) radius 1.1
  circle A174 centre (40, -56) radius 2.05
  line L524 (38.8164, -53.95) -> (41.1836, -53.95)
  line L525 (41.1836, -53.95) -> (42.3671, -56)
  line L526 (42.3671, -56) -> (41.1836, -58.05)
  line L527 (41.1836, -58.05) -> (38.8164, -58.05)
  line L528 (38.8164, -58.05) -> (37.6329, -56)
  line L529 (37.6329, -56) -> (38.8164, -53.95)
  circle A175 centre (40, -56) radius 1.1
  circle A176 centre (40, -64) radius 2.05
  line L530 (38.8164, -61.95) -> (41.1836, -61.95)
  line L531 (41.1836, -61.95) -> (42.3671, -64)
  line L532 (42.3671, -64) -> (41.1836, -66.05)
  line L533 (41.1836, -66.05) -> (38.8164, -66.05)
  line L534 (38.8164, -66.05) -> (37.6329, -64)
  line L535 (37.6329, -64) -> (38.8164, -61.95)
  circle A177 centre (40, -64) radius 1.1
  circle A178 centre (40, -72) radius 2.05
  line L536 (38.8164, -69.95) -> (41.1836, -69.95)
  line L537 (41.1836, -69.95) -> (42.3671, -72)
  line L538 (42.3671, -72) -> (41.1836, -74.05)
  line L539 (41.1836, -74.05) -> (38.8164, -74.05)
  line L540 (38.8164, -74.05) -> (37.6329, -72)
  line L541 (37.6329, -72) -> (38.8164, -69.95)
  circle A179 centre (40, -72) radius 1.1
  circle A180 centre (40, -80) radius 2.05
  line L542 (38.8164, -77.95) -> (41.1836, -77.95)
  line L543 (41.1836, -77.95) -> (42.3671, -80)
  line L544 (42.3671, -80) -> (41.1836, -82.05)
  line L545 (41.1836, -82.05) -> (38.8164, -82.05)
  line L546 (38.8164, -82.05) -> (37.6329, -80)
  line L547 (37.6329, -80) -> (38.8164, -77.95)
  circle A181 centre (40, -80) radius 1.1
  circle A182 centre (40, -88) radius 2.05
  line L548 (38.8164, -85.95) -> (41.1836, -85.95)
  line L549 (41.1836, -85.95) -> (42.3671, -88)
  line L550 (42.3671, -88) -> (41.1836, -90.05)
  line L551 (41.1836, -90.05) -> (38.8164, -90.05)
  line L552 (38.8164, -90.05) -> (37.6329, -88)
  line L553 (37.6329, -88) -> (38.8164, -85.95)
  circle A183 centre (40, -88) radius 1.1
  circle A184 centre (40, -96) radius 2.05
  line L554 (38.8164, -93.95) -> (41.1836, -93.95)
  line L555 (41.1836, -93.95) -> (42.3671, -96)
  line L556 (42.3671, -96) -> (41.1836, -98.05)
  line L557 (41.1836, -98.05) -> (38.8164, -98.05)
  line L558 (38.8164, -98.05) -> (37.6329, -96)
  line L559 (37.6329, -96) -> (38.8164, -93.95)
  circle A185 centre (40, -96) radius 1.1
  circle A186 centre (40, -104) radius 2.05
  line L560 (38.8164, -101.95) -> (41.1836, -101.95)
  line L561 (41.1836, -101.95) -> (42.3671, -104)
  line L562 (42.3671, -104) -> (41.1836, -106.05)
  line L563 (41.1836, -106.05) -> (38.8164, -106.05)
  line L564 (38.8164, -106.05) -> (37.6329, -104)
  line L565 (37.6329, -104) -> (38.8164, -101.95)
  circle A187 centre (40, -104) radius 1.1
  circle A188 centre (40, -112) radius 2.05
  line L566 (38.8164, -109.95) -> (41.1836, -109.95)
  line L567 (41.1836, -109.95) -> (42.3671, -112)
  line L568 (42.3671, -112) -> (41.1836, -114.05)
  line L569 (41.1836, -114.05) -> (38.8164, -114.05)
  line L570 (38.8164, -114.05) -> (37.6329, -112)
  line L571 (37.6329, -112) -> (38.8164, -109.95)
  circle A189 centre (40, -112) radius 1.1
  circle A190 centre (40, -120) radius 2.05
  line L572 (38.8164, -117.95) -> (41.1836, -117.95)
  line L573 (41.1836, -117.95) -> (42.3671, -120)
  line L574 (42.3671, -120) -> (41.1836, -122.05)
  line L575 (41.1836, -122.05) -> (38.8164, -122.05)
  line L576 (38.8164, -122.05) -> (37.6329, -120)
  line L577 (37.6329, -120) -> (38.8164, -117.95)
  circle A191 centre (40, -120) radius 1.1
  circle A192 centre (48, 0) radius 2.05
  line L578 (46.8164, 2.05) -> (49.1836, 2.05)
  line L579 (49.1836, 2.05) -> (50.3671, 0)
  line L580 (50.3671, 0) -> (49.1836, -2.05)
  line L581 (49.1836, -2.05) -> (46.8164, -2.05)
  line L582 (46.8164, -2.05) -> (45.6329, 0)
  line L583 (45.6329, 0) -> (46.8164, 2.05)
  circle A193 centre (48, 0) radius 1.1
  circle A194 centre (48, -8) radius 2.05
  line L584 (46.8164, -5.95) -> (49.1836, -5.95)
  line L585 (49.1836, -5.95) -> (50.3671, -8)
  line L586 (50.3671, -8) -> (49.1836, -10.05)
  line L587 (49.1836, -10.05) -> (46.8164, -10.05)
  line L588 (46.8164, -10.05) -> (45.6329, -8)
  line L589 (45.6329, -8) -> (46.8164, -5.95)
  circle A195 centre (48, -8) radius 1.1
  circle A196 centre (48, -16) radius 2.05
  line L590 (46.8164, -13.95) -> (49.1836, -13.95)
  line L591 (49.1836, -13.95) -> (50.3671, -16)
  line L592 (50.3671, -16) -> (49.1836, -18.05)
  line L593 (49.1836, -18.05) -> (46.8164, -18.05)
  line L594 (46.8164, -18.05) -> (45.6329, -16)
  line L595 (45.6329, -16) -> (46.8164, -13.95)
  circle A197 centre (48, -16) radius 1.1
  circle A198 centre (48, -24) radius 2.05
  line L596 (46.8164, -21.95) -> (49.1836, -21.95)
  line L597 (49.1836, -21.95) -> (50.3671, -24)
  line L598 (50.3671, -24) -> (49.1836, -26.05)
  line L599 (49.1836, -26.05) -> (46.8164, -26.05)
  line L600 (46.8164, -26.05) -> (45.6329, -24)
  line L601 (45.6329, -24) -> (46.8164, -21.95)
  circle A199 centre (48, -24) radius 1.1
  circle A200 centre (48, -32) radius 2.05
  line L602 (46.8164, -29.95) -> (49.1836, -29.95)
  line L603 (49.1836, -29.95) -> (50.3671, -32)
  line L604 (50.3671, -32) -> (49.1836, -34.05)
  line L605 (49.1836, -34.05) -> (46.8164, -34.05)
  line L606 (46.8164, -34.05) -> (45.6329, -32)
  line L607 (45.6329, -32) -> (46.8164, -29.95)
  circle A201 centre (48, -32) radius 1.1
  circle A202 centre (48, -40) radius 2.05
  line L608 (46.8164, -37.95) -> (49.1836, -37.95)
  line L609 (49.1836, -37.95) -> (50.3671, -40)
  line L610 (50.3671, -40) -> (49.1836, -42.05)
  line L611 (49.1836, -42.05) -> (46.8164, -42.05)
  line L612 (46.8164, -42.05) -> (45.6329, -40)
  line L613 (45.6329, -40) -> (46.8164, -37.95)
  circle A203 centre (48, -40) radius 1.1
  circle A204 centre (48, -48) radius 2.05
  line L614 (46.8164, -45.95) -> (49.1836, -45.95)
  line L615 (49.1836, -45.95) -> (50.3671, -48)
  line L616 (50.3671, -48) -> (49.1836, -50.05)
  line L617 (49.1836, -50.05) -> (46.8164, -50.05)
  line L618 (46.8164, -50.05) -> (45.6329, -48)
  line L619 (45.6329, -48) -> (46.8164, -45.95)
  circle A205 centre (48, -48) radius 1.1
  circle A206 centre (48, -56) radius 2.05
  line L620 (46.8164, -53.95) -> (49.1836, -53.95)
  line L621 (49.1836, -53.95) -> (50.3671, -56)
  line L622 (50.3671, -56) -> (49.1836, -58.05)
  line L623 (49.1836, -58.05) -> (46.8164, -58.05)
  line L624 (46.8164, -58.05) -> (45.6329, -56)
  line L625 (45.6329, -56) -> (46.8164, -53.95)
  circle A207 centre (48, -56) radius 1.1
  circle A208 centre (48, -64) radius 2.05
  line L626 (46.8164, -61.95) -> (49.1836, -61.95)
  line L627 (49.1836, -61.95) -> (50.3671, -64)
  line L628 (50.3671, -64) -> (49.1836, -66.05)
  line L629 (49.1836, -66.05) -> (46.8164, -66.05)
  line L630 (46.8164, -66.05) -> (45.6329, -64)
  line L631 (45.6329, -64) -> (46.8164, -61.95)
  circle A209 centre (48, -64) radius 1.1
  circle A210 centre (48, -72) radius 2.05
  line L632 (46.8164, -69.95) -> (49.1836, -69.95)
  line L633 (49.1836, -69.95) -> (50.3671, -72)
  line L634 (50.3671, -72) -> (49.1836, -74.05)
  line L635 (49.1836, -74.05) -> (46.8164, -74.05)
  line L636 (46.8164, -74.05) -> (45.6329, -72)
  line L637 (45.6329, -72) -> (46.8164, -69.95)
  circle A211 centre (48, -72) radius 1.1
  circle A212 centre (48, -80) radius 2.05
  line L638 (46.8164, -77.95) -> (49.1836, -77.95)
  line L639 (49.1836, -77.95) -> (50.3671, -80)
  line L640 (50.3671, -80) -> (49.1836, -82.05)
  line L641 (49.1836, -82.05) -> (46.8164, -82.05)
  line L642 (46.8164, -82.05) -> (45.6329, -80)
  line L643 (45.6329, -80) -> (46.8164, -77.95)
  circle A213 centre (48, -80) radius 1.1
  circle A214 centre (48, -88) radius 2.05
  line L644 (46.8164, -85.95) -> (49.1836, -85.95)
  line L645 (49.1836, -85.95) -> (50.3671, -88)
  line L646 (50.3671, -88) -> (49.1836, -90.05)
  line L647 (49.1836, -90.05) -> (46.8164, -90.05)
  line L648 (46.8164, -90.05) -> (45.6329, -88)
  line L649 (45.6329, -88) -> (46.8164, -85.95)
  circle A215 centre (48, -88) radius 1.1
  circle A216 centre (48, -96) radius 2.05
  line L650 (46.8164, -93.95) -> (49.1836, -93.95)
  line L651 (49.1836, -93.95) -> (50.3671, -96)
  line L652 (50.3671, -96) -> (49.1836, -98.05)
  line L653 (49.1836, -98.05) -> (46.8164, -98.05)
  line L654 (46.8164, -98.05) -> (45.6329, -96)
  line L655 (45.6329, -96) -> (46.8164, -93.95)
  circle A217 centre (48, -96) radius 1.1
  circle A218 centre (48, -104) radius 2.05
  line L656 (46.8164, -101.95) -> (49.1836, -101.95)
  line L657 (49.1836, -101.95) -> (50.3671, -104)
  line L658 (50.3671, -104) -> (49.1836, -106.05)
  line L659 (49.1836, -106.05) -> (46.8164, -106.05)
  line L660 (46.8164, -106.05) -> (45.6329, -104)
  line L661 (45.6329, -104) -> (46.8164, -101.95)
  circle A219 centre (48, -104) radius 1.1
  circle A220 centre (48, -112) radius 2.05
  line L662 (46.8164, -109.95) -> (49.1836, -109.95)
  line L663 (49.1836, -109.95) -> (50.3671, -112)
  line L664 (50.3671, -112) -> (49.1836, -114.05)
  line L665 (49.1836, -114.05) -> (46.8164, -114.05)
  line L666 (46.8164, -114.05) -> (45.6329, -112)
  line L667 (45.6329, -112) -> (46.8164, -109.95)
  circle A221 centre (48, -112) radius 1.1
  circle A222 centre (48, -120) radius 2.05
  line L668 (46.8164, -117.95) -> (49.1836, -117.95)
  line L669 (49.1836, -117.95) -> (50.3671, -120)
  line L670 (50.3671, -120) -> (49.1836, -122.05)
  line L671 (49.1836, -122.05) -> (46.8164, -122.05)
  line L672 (46.8164, -122.05) -> (45.6329, -120)
  line L673 (45.6329, -120) -> (46.8164, -117.95)
  circle A223 centre (48, -120) radius 1.1
  circle A224 centre (56, 0) radius 2.05
  line L674 (54.8164, 2.05) -> (57.1836, 2.05)
  line L675 (57.1836, 2.05) -> (58.3671, 0)
  line L676 (58.3671, 0) -> (57.1836, -2.05)
  line L677 (57.1836, -2.05) -> (54.8164, -2.05)
  line L678 (54.8164, -2.05) -> (53.6329, 0)
  line L679 (53.6329, 0) -> (54.8164, 2.05)
  circle A225 centre (56, 0) radius 1.1
  circle A226 centre (56, -8) radius 2.05
  line L680 (54.8164, -5.95) -> (57.1836, -5.95)
  line L681 (57.1836, -5.95) -> (58.3671, -8)
  line L682 (58.3671, -8) -> (57.1836, -10.05)
  line L683 (57.1836, -10.05) -> (54.8164, -10.05)
  line L684 (54.8164, -10.05) -> (53.6329, -8)
  line L685 (53.6329, -8) -> (54.8164, -5.95)
  circle A227 centre (56, -8) radius 1.1
  circle A228 centre (56, -16) radius 2.05
  line L686 (54.8164, -13.95) -> (57.1836, -13.95)
  line L687 (57.1836, -13.95) -> (58.3671, -16)
  line L688 (58.3671, -16) -> (57.1836, -18.05)
  line L689 (57.1836, -18.05) -> (54.8164, -18.05)
  line L690 (54.8164, -18.05) -> (53.6329, -16)
  line L691 (53.6329, -16) -> (54.8164, -13.95)
  circle A229 centre (56, -16) radius 1.1
  circle A230 centre (56, -24) radius 2.05
  line L692 (54.8164, -21.95) -> (57.1836, -21.95)
  line L693 (57.1836, -21.95) -> (58.3671, -24)
  line L694 (58.3671, -24) -> (57.1836, -26.05)
  line L695 (57.1836, -26.05) -> (54.8164, -26.05)
  line L696 (54.8164, -26.05) -> (53.6329, -24)
  line L697 (53.6329, -24) -> (54.8164, -21.95)
  circle A231 centre (56, -24) radius 1.1
  circle A232 centre (56, -32) radius 2.05
  line L698 (54.8164, -29.95) -> (57.1836, -29.95)
  line L699 (57.1836, -29.95) -> (58.3671, -32)
  line L700 (58.3671, -32) -> (57.1836, -34.05)
  line L701 (57.1836, -34.05) -> (54.8164, -34.05)
  line L702 (54.8164, -34.05) -> (53.6329, -32)
  line L703 (53.6329, -32) -> (54.8164, -29.95)
  circle A233 centre (56, -32) radius 1.1
  circle A234 centre (56, -40) radius 2.05
  line L704 (54.8164, -37.95) -> (57.1836, -37.95)
  line L705 (57.1836, -37.95) -> (58.3671, -40)
  line L706 (58.3671, -40) -> (57.1836, -42.05)
  line L707 (57.1836, -42.05) -> (54.8164, -42.05)
  line L708 (54.8164, -42.05) -> (53.6329, -40)
  line L709 (53.6329, -40) -> (54.8164, -37.95)
  circle A235 centre (56, -40) radius 1.1
  circle A236 centre (56, -48) radius 2.05
  line L710 (54.8164, -45.95) -> (57.1836, -45.95)
  line L711 (57.1836, -45.95) -> (58.3671, -48)
  line L712 (58.3671, -48) -> (57.1836, -50.05)
  line L713 (57.1836, -50.05) -> (54.8164, -50.05)
  line L714 (54.8164, -50.05) -> (53.6329, -48)
  line L715 (53.6329, -48) -> (54.8164, -45.95)
  circle A237 centre (56, -48) radius 1.1
  circle A238 centre (56, -56) radius 2.05
  line L716 (54.8164, -53.95) -> (57.1836, -53.95)
  line L717 (57.1836, -53.95) -> (58.3671, -56)
  line L718 (58.3671, -56) -> (57.1836, -58.05)
  line L719 (57.1836, -58.05) -> (54.8164, -58.05)
  line L720 (54.8164, -58.05) -> (53.6329, -56)
  line L721 (53.6329, -56) -> (54.8164, -53.95)
  circle A239 centre (56, -56) radius 1.1
  circle A240 centre (56, -64) radius 2.05
  line L722 (54.8164, -61.95) -> (57.1836, -61.95)
  line L723 (57.1836, -61.95) -> (58.3671, -64)
  line L724 (58.3671, -64) -> (57.1836, -66.05)
  line L725 (57.1836, -66.05) -> (54.8164, -66.05)
  line L726 (54.8164, -66.05) -> (53.6329, -64)
  line L727 (53.6329, -64) -> (54.8164, -61.95)
  circle A241 centre (56, -64) radius 1.1
  circle A242 centre (56, -72) radius 2.05
  line L728 (54.8164, -69.95) -> (57.1836, -69.95)
  line L729 (57.1836, -69.95) -> (58.3671, -72)
  line L730 (58.3671, -72) -> (57.1836, -74.05)
  line L731 (57.1836, -74.05) -> (54.8164, -74.05)
  line L732 (54.8164, -74.05) -> (53.6329, -72)
  line L733 (53.6329, -72) -> (54.8164, -69.95)
  circle A243 centre (56, -72) radius 1.1
  circle A244 centre (56, -80) radius 2.05
  line L734 (54.8164, -77.95) -> (57.1836, -77.95)
  line L735 (57.1836, -77.95) -> (58.3671, -80)
  line L736 (58.3671, -80) -> (57.1836, -82.05)
  line L737 (57.1836, -82.05) -> (54.8164, -82.05)
  line L738 (54.8164, -82.05) -> (53.6329, -80)
  line L739 (53.6329, -80) -> (54.8164, -77.95)
  circle A245 centre (56, -80) radius 1.1
  circle A246 centre (56, -88) radius 2.05
  line L740 (54.8164, -85.95) -> (57.1836, -85.95)
  line L741 (57.1836, -85.95) -> (58.3671, -88)
  line L742 (58.3671, -88) -> (57.1836, -90.05)
  line L743 (57.1836, -90.05) -> (54.8164, -90.05)
  line L744 (54.8164, -90.05) -> (53.6329, -88)
  line L745 (53.6329, -88) -> (54.8164, -85.95)
  circle A247 centre (56, -88) radius 1.1
  circle A248 centre (56, -96) radius 2.05
  line L746 (54.8164, -93.95) -> (57.1836, -93.95)
  line L747 (57.1836, -93.95) -> (58.3671, -96)
  line L748 (58.3671, -96) -> (57.1836, -98.05)
  line L749 (57.1836, -98.05) -> (54.8164, -98.05)
  line L750 (54.8164, -98.05) -> (53.6329, -96)
  line L751 (53.6329, -96) -> (54.8164, -93.95)
  circle A249 centre (56, -96) radius 1.1
  circle A250 centre (56, -104) radius 2.05
  line L752 (54.8164, -101.95) -> (57.1836, -101.95)
  line L753 (57.1836, -101.95) -> (58.3671, -104)
  line L754 (58.3671, -104) -> (57.1836, -106.05)
  line L755 (57.1836, -106.05) -> (54.8164, -106.05)
  line L756 (54.8164, -106.05) -> (53.6329, -104)
  line L757 (53.6329, -104) -> (54.8164, -101.95)
  circle A251 centre (56, -104) radius 1.1
  circle A252 centre (56, -112) radius 2.05
  line L758 (54.8164, -109.95) -> (57.1836, -109.95)
  line L759 (57.1836, -109.95) -> (58.3671, -112)
  line L760 (58.3671, -112) -> (57.1836, -114.05)
  line L761 (57.1836, -114.05) -> (54.8164, -114.05)
  line L762 (54.8164, -114.05) -> (53.6329, -112)
  line L763 (53.6329, -112) -> (54.8164, -109.95)
  circle A253 centre (56, -112) radius 1.1
  circle A254 centre (56, -120) radius 2.05
  line L764 (54.8164, -117.95) -> (57.1836, -117.95)
  line L765 (57.1836, -117.95) -> (58.3671, -120)
  line L766 (58.3671, -120) -> (57.1836, -122.05)
  line L767 (57.1836, -122.05) -> (54.8164, -122.05)
  line L768 (54.8164, -122.05) -> (53.6329, -120)
  line L769 (53.6329, -120) -> (54.8164, -117.95)
  circle A255 centre (56, -120) radius 1.1
  circle A256 centre (64, 0) radius 2.05
  line L770 (62.8164, 2.05) -> (65.1836, 2.05)
  line L771 (65.1836, 2.05) -> (66.3671, 0)
  line L772 (66.3671, 0) -> (65.1836, -2.05)
  line L773 (65.1836, -2.05) -> (62.8164, -2.05)
  line L774 (62.8164, -2.05) -> (61.6329, 0)
  line L775 (61.6329, 0) -> (62.8164, 2.05)
  circle A257 centre (64, 0) radius 1.1
  circle A258 centre (64, -8) radius 2.05
  line L776 (62.8164, -5.95) -> (65.1836, -5.95)
  line L777 (65.1836, -5.95) -> (66.3671, -8)
  line L778 (66.3671, -8) -> (65.1836, -10.05)
  line L779 (65.1836, -10.05) -> (62.8164, -10.05)
  line L780 (62.8164, -10.05) -> (61.6329, -8)
  line L781 (61.6329, -8) -> (62.8164, -5.95)
  circle A259 centre (64, -8) radius 1.1
  circle A260 centre (64, -16) radius 2.05
  line L782 (62.8164, -13.95) -> (65.1836, -13.95)
  line L783 (65.1836, -13.95) -> (66.3671, -16)
  line L784 (66.3671, -16) -> (65.1836, -18.05)
  line L785 (65.1836, -18.05) -> (62.8164, -18.05)
  line L786 (62.8164, -18.05) -> (61.6329, -16)
  line L787 (61.6329, -16) -> (62.8164, -13.95)
  circle A261 centre (64, -16) radius 1.1
  circle A262 centre (64, -24) radius 2.05
  line L788 (62.8164, -21.95) -> (65.1836, -21.95)
  line L789 (65.1836, -21.95) -> (66.3671, -24)